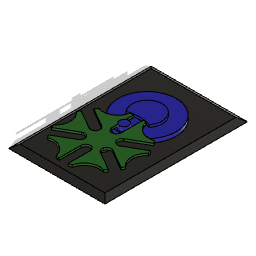
Geneva Mechanism (Autodesk Fusion 360 design; units mm, degrees)
Autodesk Fusion 360 part; units mm, degrees
sketch "holder bottom" plane through (0, 0, 0) normal (0, 0, 1) x (1, 0, 0) in component "holder"
  line L0 (-92.5, 62.5) -> (92.5, 62.5)
  line L1 (92.5, 62.5) -> (92.5, -62.5)
  line L2 (92.5, -62.5) -> (-92.5, -62.5)
  line L3 (-92.5, -62.5) -> (-92.5, 62.5)
  line L4 (-92.5, 62.5) -> (92.5, -62.5) construction
  line L5 (92.5, 62.5) -> (-92.5, -62.5) construction
  dimension "d7" = 185
  dimension "d8" = 125
  constraint horizontal L0
  constraint perpendicular L0 L1
  constraint parallel L0 L2
  constraint parallel L1 L3
  constraint coincident L4 origin
  constraint coincident L5 origin
  measures "d7" distance of L0.start L0.end
  measures "d8" distance of L0.start L2.end
ref_plane "WorkPlane1" through (0, 0, 5) normal (0, 0, 1) x (1, 0, 0) in component "holder"
sketch "holder top" plane through (0, 0, 5) normal (0, 0, 1) x (1, 0, 0) in component "holder"
  line L0 (-85, 55) -> (85, 55)
  line L1 (85, 55) -> (85, -55)
  line L2 (85, -55) -> (-85, -55)
  line L3 (-85, -55) -> (-85, 55)
  line L4 (-85, 55) -> (85, -55) construction
  line L5 (85, 55) -> (-85, -55) construction
  circle A0 centre (-25, 0) radius 7.5
  circle A1 centre (35, 0) radius 7.5
  dimension "d9" = 170
  dimension "d10" = 110
  dimension "d11" = 15
  dimension "d12" = 15
  constraint horizontal L0
  constraint perpendicular L0 L1
  constraint parallel L0 L2
  constraint parallel L1 L3
  constraint coincident L4 origin
  constraint coincident L5 origin
  measures "d9" distance of L0.start L0.end
  measures "d10" distance of L0.start L2.end
  measures "d11" diameter of A0
  measures "d12" diameter of A1
loft "Loft1" add profiles "holder top", "holder bottom" section 1 contours L0 L1 L2 L3 | A0 | A1 section 2 makes body 1 in component "holder"
extrude "Extrude2" cut sketch "holder top" against normal blind 15 contours A0 | A1 bodies 1 in component "holder"
sketch "drive wheel" plane through (0, 0, 5) normal (0, 0, 1) x (1, 0, 0) in component "drive wheel"
  circle A0 centre (-25, 0) radius 6.5
  circle A1 centre (-25, 0) radius 37.5
  circle A2 centre (-25, 0) radius 20
  dimension "d15" = 13
  dimension "d16" = 75
  dimension "d21" = 40
  constraint concentric A0 A1
  constraint concentric A1 A2
  measures "d15" diameter of A0
  measures "d16" diameter of A1
  measures "d21" diameter of A2
extrude "Extrude1" add sketch "drive wheel" against normal blind 5 separate body contours A0 makes body 2 in component "drive wheel"
extrude "Extrude2'" add sketch "drive wheel" along normal blind 5 separate body contours A1 | A2 makes body 3 in component "drive wheel"
extrude "Extrude3" add sketch "drive wheel" along normal blind 8 contours A0 | A2 bodies 3 2 in component "drive wheel"
sketch "drivel wheel" plane through (0, 0, 5) normal (0, 0, 1) x (1, 0, 0) in component "driven wheel"
  circle A0 centre (35, 0) radius 49.9
  circle A1 centre (35, 0) radius 6.5
  circle A2 centre (35, 0) radius 10
  dimension "d24" = 99.8
  dimension "d25" = 13
  constraint concentric A0 A1
  constraint concentric A0 A2
  measures "d24" diameter of A0
  measures "d25" diameter of A1
extrude "Extrude1'" add sketch "drivel wheel" against normal blind 5 separate body contours A1 makes body 4 in component "driven wheel"
extrude "Extrude2''" add sketch "drivel wheel" along normal blind 5.3 contours A1 | A2 bodies 4 in component "driven wheel"
extrude "Extrude4" cut sketch "drivel wheel" along normal blind 8 and the other way blind -5 contours A0 bodies 3 in component "drive wheel"
extrude "Extrude3'" add sketch "drivel wheel" along normal blind 8 and the other way blind -5.3 contours A0 | A1 | A2 bodies 4 in component "driven wheel"
sketch "half circle cut" plane through (0, 0, 13) normal (0, 0, 1) x (-1, 0, 0) in component "driven wheel"
  circle A0 centre (-35, 0) radius 49.9
  circle A1 centre (25, 0) radius 20
  dimension "d38" = 40
  measures "d38" diameter of A1
extrude "Extrude4'" cut sketch "half circle cut" against normal blind 3 contours A0 A1 picked at (11.5806, -2.7389) bodies 4 in component "driven wheel"
pattern_circular "C-Pattern1" count 6 over 360 about axis through (35, 0, 13) along (0, 0, 1) of "Extrude4'" in component "driven wheel"
move_face "OffsetFaces1" offset 0.8 1 faces at (41.4677, -0.6472, 3.3333) on bodies 4 in component "driven wheel"
move_face "OffsetFaces1'" offset 0.8 1 faces at (-18.5323, -0.6472, 3.3333) on bodies 3 in component "drive wheel"
sketch "elongated cut" plane through (0, 0, 13) normal (0, 0, 1) x (-1, 0, 0) in component "driven wheel"
  arc A0 (2.1712, -33.2914) -> (-24.7544, -48.8368) centre (-5, -51.9615) ccw
  arc A1 (2.1712, -33.2914) -> (12.4167, -15.5455) centre (-35, 0) ccw
  arc A2 (12.4167, 15.5455) -> (12.4167, -15.5455) centre (25, 0) ccw
  arc A3 (12.4167, 15.5455) -> (2.1712, 33.2914) centre (-35, 0) ccw
  arc A4 (-24.7544, 48.8368) -> (2.1712, 33.2914) centre (-5, 51.9615) ccw
  arc A5 (-24.7544, 48.8368) -> (-45.2456, 48.8368) centre (-35, 0) ccw
  arc A6 (-72.1712, 33.2914) -> (-45.2456, 48.8368) centre (-65, 51.9615) ccw
  arc A7 (-72.1712, 33.2914) -> (-82.4168, 15.5455) centre (-35, 0) ccw
  arc A8 (-82.4168, -15.5455) -> (-82.4168, 15.5455) centre (-95, 0) ccw
  arc A9 (-82.4168, -15.5455) -> (-72.1712, -33.2914) centre (-35, 0) ccw
  arc A10 (-45.2456, -48.8368) -> (-72.1712, -33.2914) centre (-65, -51.9615) ccw
  arc A11 (-45.2456, -48.8368) -> (-24.7544, -48.8368) centre (-35, 0) ccw
  line L0 (-41.032, -48.7029) -> (-41.0102, -19.9954)
  line L1 (-29.0092, -48.9425) -> (-29.0102, -20.0007)
  line L2 (-29.0092, -48.9425) -> (-29.0093, -49.5391)
  line L3 (-41.032, -48.7029) -> (-41.0325, -49.534)
  arc A12 (-29.0102, -20.0007) -> (-41.0102, -19.9954) centre (-35.0102, -20) ccw
  line L4 (10.3808, -19.283) -> (-14.684, -4.813)
  line L5 (4.1619, -29.5753) -> (-20.6885, -15.2027)
  arc A13 (-14.684, -4.813) -> (-20.6885, -15.2027) centre (-17.6846, -10.0088) ccw
  line L6 (10.3808, -19.283) -> (10.8975, -19.5814)
  line L7 (4.1619, -29.5753) -> (4.8815, -29.9913)
  line L8 (4.39, 29.6594) -> (-20.6738, 15.1877)
  line L9 (10.194, 19.1275) -> (-14.6784, 4.7927)
  arc A14 (-20.6738, 15.1877) -> (-14.6784, 4.7927) centre (-17.6744, 9.9912) ccw
  line L10 (4.39, 29.6594) -> (4.9068, 29.9576)
  line L11 (10.194, 19.1275) -> (10.9139, 19.5428)
  line L12 (-40.9908, 48.9425) -> (-40.9898, 20.0007)
  line L13 (-28.968, 48.7029) -> (-28.9898, 19.9954)
  arc A15 (-40.9898, 20.0007) -> (-28.9898, 19.9954) centre (-34.9898, 20) ccw
  line L14 (-40.9908, 48.9425) -> (-40.9907, 49.5391)
  line L15 (-28.968, 48.7029) -> (-28.9675, 49.534)
  line L16 (-80.3808, 19.283) -> (-55.316, 4.813)
  line L17 (-74.1619, 29.5753) -> (-49.3115, 15.2027)
  arc A16 (-55.316, 4.813) -> (-49.3115, 15.2027) centre (-52.3154, 10.0088) ccw
  line L18 (-80.3808, 19.283) -> (-80.8975, 19.5814)
  line L19 (-74.1619, 29.5753) -> (-74.8815, 29.9913)
  line L20 (-74.39, -29.6594) -> (-49.3262, -15.1877)
  line L21 (-80.194, -19.1275) -> (-55.3216, -4.7927)
  arc A17 (-49.3262, -15.1877) -> (-55.3216, -4.7927) centre (-52.3256, -9.9912) ccw
  line L22 (-74.39, -29.6594) -> (-74.9068, -29.9576)
  line L23 (-80.194, -19.1275) -> (-80.9139, -19.5428)
  dimension "d54" = 20
  dimension "d55" = 12
  dimension "d57" = 360
  constraint tangent L0 A12
  constraint coincident A11 L2.end
  constraint coincident A11 L3.end
  measures "d54" distance of A1.centre A12.centre
  measures "d55" diameter of A12
extrude "Extrude5" cut sketch "elongated cut" against normal blind 2.7 contours A1 L4 L5 A13 L6 L7 | A11 L0 L1 L2 L3 A12 | A3 L8 L9 A14 L10 L11 | A9 L20 L21 A17 L22 L23 | A5 L12 L13 A15 L14 L15 | A7 L16 L17 A16 L18 L19 bodies 4 in component "driven wheel"
sketch "pin" plane through (0, 0, 10) normal (0, 0, 1) x (-1, 0, 0)
  arc A0 (12.4167, -15.5455) -> (12.4167, 15.5455) centre (25, 0) ccw
  arc A1 (12.4167, -15.5455) -> (12.4167, 15.5455) centre (-35, 0) ccw
  circle A2 centre (25, 0) radius 37.5
  line L0 (25, 0) -> (-5, 0)
  circle A3 centre (-5, 0) radius 6
  dimension "d79" = 12
  constraint coincident A0.centre A2.centre
  constraint horizontal L0
  constraint coincident L0.end A3.centre
  measures "d79" diameter of A3
extrude "Extrude7" add sketch "pin" along normal blind 6 contours A3 bodies 3 in component "drive wheel"
sketch "offset" plane through (0, 0, 5) normal (0, 0, 1) x (1, 0, 0) in component "drive wheel"
  circle A0 centre (35, 0) radius 50
  circle A1 centre (35, 0) radius 49
  dimension "d82" = 100
  dimension "d83" = 98
  constraint concentric A0 A1
  measures "d82" diameter of A0
  measures "d83" diameter of A1
extrude "Extrude6" cut sketch "offset" along normal blind 15 sketch seen with x (0.000593, 1, 0) y (-1, 0.000593, 0) z (0, 0, 1) at (34.9792, -35, 0) bodies 4 in component "driven wheel"
sketch "center" plane through (0, 0, 13) normal (0, 0, 1) x (-1, 0, 0) in component "drive wheel"
  arc A0 (12.4167, -15.5455) -> (12.4167, 15.5455) centre (-35, 0) ccw
  arc A1 (12.4167, -15.5455) -> (12.4167, 15.5455) centre (25, 0) ccw
  circle A2 centre (25, 0) radius 19.5
  dimension "d86" = 39
  constraint concentric A1 A2
  measures "d86" diameter of A2
extrude "Extrude8" cut sketch "center" against normal blind 3 contours A0 A1 A2 bodies 3 in component "drive wheel"
component "holder" placed x (1, 0, 0) y (0, 1, 0) z (0, 0, 1) at (0, 0, 0)
component "drive wheel" placed x (1, 0, 0) y (0, 1, 0) z (0, 0, 1) at (0, 0, 0)
component "driven wheel" placed x (0.000593, -1, 0) y (1, 0.000593, 0) z (0, 0, 1) at (34.9792, 35, 0)
named bodies: "holder", "drive wheel", "driven wheel"
